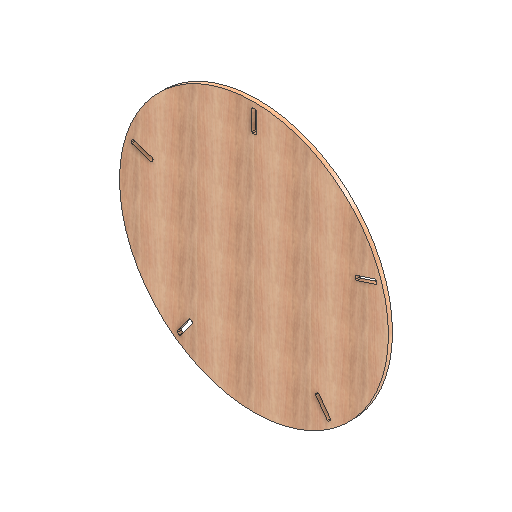
# Autodesk Inventor part: Disk G
Saved by Autodesk Inventor 2021 (Build 250183000, 183)
## iProperties
Created: 2020-05-09
Part Number: Disk G
Material: Wood (Birch)
Document SubType Name: Modeling
Designer: Dan Wikman
Density: 0.55 g/cm^3
Appearance: Birch - Natural Polished
Mass: 11105 g
Surface Area: 23317.4 cm^2
Volume: 20191 cm^3
Autodesk Inventor part; units mm, degrees
ref_plane "YZ Plane" through (0, 0, 0) normal (1, 0, 0) x (0, 1, 0)
ref_plane "XZ Plane" through (0, 0, 0) normal (0, 1, 0) x (-1, 0, 0)
ref_plane "XY Plane" through (0, 0, 0) normal (0, 0, 1) x (1, 0, 0)
sketch "CONTOURS" plane through (0, 0, 0) normal (0, 0, 1) x (1, 0, 0)
  circle A0 centre (614.9903, 609.9576) radius 599.9973
  dimension "d3" = 1199.9946
  constraints: 1 centre point
  measures "d3" diameter of A0
sketch "HOLES" plane through (0, 0, 0) normal (0, 0, 1) x (1, 0, 0)
  line L0 (1162.6152, 782.0631) -> (1159.216, 792.5247)
  arc A0 (1159.216, 792.5247) -> (1154.1757, 795.0928) centre (1155.4118, 791.2886) ccw
  line L1 (1154.1757, 795.0928) -> (1068.5806, 767.2813)
  arc A1 (1068.5806, 767.2813) -> (1066.0124, 762.241) centre (1069.8167, 763.4771) ccw
  line L2 (1066.0124, 762.241) -> (1069.4116, 751.7794)
  arc A2 (1069.4116, 751.7794) -> (1074.4519, 749.2112) centre (1073.2159, 753.0155) ccw
  line L3 (1074.4519, 749.2112) -> (1160.047, 777.0228)
  arc A3 (1160.047, 777.0228) -> (1162.6152, 782.0631) centre (1158.8109, 780.827) ccw
  line L4 (947.8978, 142.3189) -> (956.7969, 148.7846)
  arc A4 (956.7969, 148.7846) -> (957.6819, 154.3718) centre (954.4458, 152.0206) ccw
  line L5 (957.6819, 154.3718) -> (904.7812, 227.1833)
  arc A5 (904.7812, 227.1833) -> (899.194, 228.0682) centre (901.5451, 224.8322) ccw
  line L6 (899.194, 228.0682) -> (890.2948, 221.6026)
  arc A6 (890.2948, 221.6026) -> (889.4099, 216.0154) centre (892.6459, 218.3665) ccw
  line L7 (889.4099, 216.0154) -> (942.3106, 143.2039)
  arc A7 (942.3106, 143.2039) -> (947.8978, 142.3189) centre (945.5466, 145.555) ccw
  line L8 (620.5337, 1183.9633) -> (609.5337, 1183.9633)
  arc A8 (609.5337, 1183.9633) -> (605.5337, 1179.9633) centre (609.5337, 1179.9633) ccw
  line L9 (605.5337, 1179.9633) -> (605.5337, 1089.9633)
  arc A9 (605.5337, 1089.9633) -> (609.5337, 1085.9633) centre (609.5337, 1089.9633) ccw
  line L10 (609.5337, 1085.9633) -> (620.5337, 1085.9633)
  arc A10 (620.5337, 1085.9633) -> (624.5337, 1089.9633) centre (620.5337, 1089.9633) ccw
  line L11 (624.5337, 1089.9633) -> (624.5337, 1179.9633)
  arc A11 (624.5337, 1179.9633) -> (620.5337, 1183.9633) centre (620.5337, 1179.9633) ccw
  line L12 (273.1136, 148.8355) -> (282.0128, 142.3699)
  arc A12 (282.0128, 142.3699) -> (287.6, 143.2548) centre (284.3639, 145.6059) ccw
  line L13 (287.6, 143.2548) -> (340.5007, 216.0663)
  arc A13 (340.5007, 216.0663) -> (339.6157, 221.6535) centre (337.2646, 218.4175) ccw
  line L14 (339.6157, 221.6535) -> (330.7166, 228.1192)
  arc A14 (330.7166, 228.1192) -> (325.1293, 227.2342) centre (328.3654, 224.8831) ccw
  line L15 (325.1293, 227.2342) -> (272.2287, 154.4227)
  arc A15 (272.2287, 154.4227) -> (273.1136, 148.8355) centre (275.4647, 152.0716) ccw
  line L16 (70.7915, 792.6071) -> (67.3923, 782.1455)
  arc A16 (67.3923, 782.1455) -> (69.9604, 777.1052) centre (71.1965, 780.9094) ccw
  line L17 (69.9604, 777.1052) -> (155.5555, 749.2937)
  arc A17 (155.5555, 749.2937) -> (160.5958, 751.8618) centre (156.7916, 753.0979) ccw
  line L18 (160.5958, 751.8618) -> (163.995, 762.3235)
  arc A18 (163.995, 762.3235) -> (161.4268, 767.3637) centre (160.1908, 763.5595) ccw
  line L19 (161.4268, 767.3637) -> (75.8318, 795.1753)
  arc A19 (75.8318, 795.1753) -> (70.7915, 792.6071) centre (74.5957, 791.371) ccw
  dimension "d1" = 19
  dimension "d19" = 90
  constraints: 40 end point, 40 point on circle, 20 centre point
  measures "d1" distance of L9.start L11.end
  measures "d19" distance of L11.start L11.end
sketch "LETTERS" plane through (0, 0, 0) normal (0, 0, 1) x (1, 0, 0)
  line L0 (622.9768, 614.1235) -> (622.8555, 614.5546)
  line L1 (622.8555, 614.5546) -> (622.7333, 614.956)
  line L2 (622.7333, 614.956) -> (622.6101, 615.3276)
  line L3 (622.6101, 615.3276) -> (622.4861, 615.6694)
  line L4 (622.4861, 615.6694) -> (622.4237, 615.8291)
  line L5 (622.4237, 615.8291) -> (622.3611, 615.9814)
  line L6 (622.3611, 615.9814) -> (622.2982, 616.1262)
  line L7 (622.2982, 616.1262) -> (622.2351, 616.2636)
  line L8 (622.2351, 616.2636) -> (622.1718, 616.3935)
  line L9 (622.1718, 616.3935) -> (622.1083, 616.516)
  line L10 (622.1083, 616.516) -> (622.0445, 616.631)
  line L11 (622.0445, 616.631) -> (621.9805, 616.7386)
  line L12 (621.9805, 616.7386) -> (621.9154, 616.8417)
  line L13 (621.9154, 616.8417) -> (621.8484, 616.943)
  line L14 (621.8484, 616.943) -> (621.7795, 617.0428)
  line L15 (621.7795, 617.0428) -> (621.7087, 617.1408)
  line L16 (621.7087, 617.1408) -> (621.6361, 617.2373)
  line L17 (621.6361, 617.2373) -> (621.5615, 617.3321)
  line L18 (621.5615, 617.3321) -> (621.485, 617.4252)
  line L19 (621.485, 617.4252) -> (621.4066, 617.5167)
  line L20 (621.4066, 617.5167) -> (621.3264, 617.6065)
  line L21 (621.3264, 617.6065) -> (621.2442, 617.6947)
  line L22 (621.2442, 617.6947) -> (621.1602, 617.7812)
  line L23 (621.1602, 617.7812) -> (621.0742, 617.8661)
  line L24 (621.0742, 617.8661) -> (620.9864, 617.9494)
  line L25 (620.9864, 617.9494) -> (620.8966, 618.031)
  line L26 (620.8966, 618.031) -> (620.805, 618.1109)
  line L27 (620.805, 618.1109) -> (620.7115, 618.1892)
  line L28 (620.7115, 618.1892) -> (620.5209, 618.3409)
  line L29 (620.5209, 618.3409) -> (620.3269, 618.4859)
  line L30 (620.3269, 618.4859) -> (620.1297, 618.6242)
  line L31 (620.1297, 618.6242) -> (619.9292, 618.756)
  line L32 (619.9292, 618.756) -> (619.7254, 618.8811)
  line L33 (619.7254, 618.8811) -> (619.5183, 618.9995)
  line L34 (619.5183, 618.9995) -> (619.3079, 619.1114)
  line L35 (619.3079, 619.1114) -> (619.0942, 619.2166)
  line L36 (619.0942, 619.2166) -> (618.9858, 619.2666)
  line L37 (618.9858, 619.2666) -> (618.8761, 619.3148)
  line L38 (618.8761, 619.3148) -> (618.765, 619.3612)
  line L39 (618.765, 619.3612) -> (618.6526, 619.4058)
  line L40 (618.6526, 619.4058) -> (618.5388, 619.4485)
  line L41 (618.5388, 619.4485) -> (618.4237, 619.4895)
  line L42 (618.4237, 619.4895) -> (618.3072, 619.5286)
  line L43 (618.3072, 619.5286) -> (618.1894, 619.5658)
  line L44 (618.1894, 619.5658) -> (617.9497, 619.6349)
  line L45 (617.9497, 619.6349) -> (617.7046, 619.6967)
  line L46 (617.7046, 619.6967) -> (617.454, 619.7512)
  line L47 (617.454, 619.7512) -> (617.1981, 619.7984)
  line L48 (617.1981, 619.7984) -> (616.9346, 619.8392)
  line L49 (616.9346, 619.8392) -> (616.6613, 619.8746)
  line L50 (616.6613, 619.8746) -> (616.3784, 619.9045)
  line L51 (616.3784, 619.9045) -> (616.0858, 619.929)
  line L52 (616.0858, 619.929) -> (615.7835, 619.9481)
  line L53 (615.7835, 619.9481) -> (615.4715, 619.9617)
  line L54 (615.4715, 619.9617) -> (614.8184, 619.9726)
  line L55 (614.8184, 619.9726) -> (614.1719, 619.964)
  line L56 (614.1719, 619.964) -> (613.5774, 619.9385)
  line L57 (613.5774, 619.9385) -> (613.2996, 619.9194)
  line L58 (613.2996, 619.9194) -> (613.0349, 619.8959)
  line L59 (613.0349, 619.8959) -> (612.7831, 619.8683)
  line L60 (612.7831, 619.8683) -> (612.5443, 619.8364)
  line L61 (612.5443, 619.8364) -> (612.3121, 619.7985)
  line L62 (612.3121, 619.7985) -> (612.0798, 619.7532)
  line L63 (612.0798, 619.7532) -> (611.8476, 619.7002)
  line L64 (611.8476, 619.7002) -> (611.6153, 619.6397)
  line L65 (611.6153, 619.6397) -> (611.383, 619.5717)
  line L66 (611.383, 619.5717) -> (611.1508, 619.4961)
  line L67 (611.1508, 619.4961) -> (610.9185, 619.4129)
  line L68 (610.9185, 619.4129) -> (610.6862, 619.3222)
  line L69 (610.6862, 619.3222) -> (610.4529, 619.2229)
  line L70 (610.4529, 619.2229) -> (610.2174, 619.1139)
  line L71 (610.2174, 619.1139) -> (609.9798, 618.9952)
  line L72 (609.9798, 618.9952) -> (609.74, 618.8669)
  line L73 (609.74, 618.8669) -> (609.4981, 618.7289)
  line L74 (609.4981, 618.7289) -> (609.2541, 618.5813)
  line L75 (609.2541, 618.5813) -> (609.0078, 618.424)
  line L76 (609.0078, 618.424) -> (608.7595, 618.257)
  line L77 (608.7595, 618.257) -> (608.6356, 618.1697)
  line L78 (608.6356, 618.1697) -> (608.5134, 618.0797)
  line L79 (608.5134, 618.0797) -> (608.3928, 617.987)
  line L80 (608.3928, 617.987) -> (608.2739, 617.8916)
  line L81 (608.2739, 617.8916) -> (608.1567, 617.7935)
  line L82 (608.1567, 617.7935) -> (608.0411, 617.6927)
  line L83 (608.0411, 617.6927) -> (607.9272, 617.5891)
  line L84 (607.9272, 617.5891) -> (607.8149, 617.4828)
  line L85 (607.8149, 617.4828) -> (607.7043, 617.3739)
  line L86 (607.7043, 617.3739) -> (607.5953, 617.2622)
  line L87 (607.5953, 617.2622) -> (607.488, 617.1478)
  line L88 (607.488, 617.1478) -> (607.3824, 617.0307)
  line L89 (607.3824, 617.0307) -> (607.2784, 616.9108)
  line L90 (607.2784, 616.9108) -> (607.176, 616.7883)
  line L91 (607.176, 616.7883) -> (607.0754, 616.663)
  line L92 (607.0754, 616.663) -> (606.9764, 616.5351)
  line L93 (606.9764, 616.5351) -> (606.8795, 616.4051)
  line L94 (606.8795, 616.4051) -> (606.7852, 616.2738)
  line L95 (618.3393, 599.944) -> (618.5538, 599.9977)
  line L96 (618.5538, 599.9977) -> (618.7672, 600.0568)
  line L97 (618.7672, 600.0568) -> (618.9794, 600.1214)
  line L98 (618.9794, 600.1214) -> (619.1905, 600.1913)
  line L99 (619.1905, 600.1913) -> (619.4004, 600.2667)
  line L100 (619.4004, 600.2667) -> (619.6092, 600.3476)
  line L101 (619.6092, 600.3476) -> (619.8168, 600.4339)
  line L102 (619.8168, 600.4339) -> (620.0233, 600.5256)
  line L103 (620.0233, 600.5256) -> (620.2287, 600.6223)
  line L104 (620.2287, 600.6223) -> (620.4332, 600.7235)
  line L105 (620.4332, 600.7235) -> (620.6368, 600.8291)
  line L106 (620.6368, 600.8291) -> (620.8394, 600.9391)
  line L107 (620.8394, 600.9391) -> (621.0411, 601.0536)
  line L108 (621.0411, 601.0536) -> (621.2419, 601.1726)
  line L109 (621.2419, 601.1726) -> (621.4418, 601.296)
  line L110 (621.4418, 601.296) -> (621.6408, 601.4239)
  line L111 (621.6408, 601.4239) -> (622.3722, 601.9163)
  line L112 (622.3722, 601.9163) -> (622.691, 602.1415)
  line L113 (622.691, 602.1415) -> (622.9785, 602.3528)
  line L114 (622.9785, 602.3528) -> (623.4053, 602.6781)
  line L115 (623.4053, 602.6781) -> (623.5311, 602.7785)
  line L116 (623.5311, 602.7785) -> (623.572, 602.8131)
  line L117 (605.8556, 614.5967) -> (605.795, 614.4485)
  line L118 (623.587, 602.8265) -> (623.5931, 602.8322)
  line L119 (623.5931, 602.8322) -> (623.5983, 602.8373)
  line L120 (623.5983, 602.8373) -> (623.5992, 609.9994)
  line L121 (623.5992, 609.9994) -> (615.0012, 610.0005)
  line L122 (605.7369, 614.299) -> (605.5299, 613.7237)
  line L123 (605.5299, 613.7237) -> (605.4413, 613.4552)
  line L124 (605.4413, 613.4552) -> (605.3626, 613.1994)
  line L125 (605.3626, 613.1994) -> (605.294, 612.9564)
  line L126 (605.294, 612.9564) -> (605.2353, 612.7261)
  line L127 (605.2353, 612.7261) -> (605.1866, 612.5085)
  line L128 (605.1866, 612.5085) -> (605.1659, 612.4045)
  line L129 (605.1659, 612.4045) -> (605.1478, 612.3036)
  line L130 (605.1478, 612.3036) -> (605.0844, 611.8916)
  line L131 (605.0844, 611.8916) -> (605.0293, 611.4495)
  line L132 (605.0293, 611.4495) -> (604.9825, 610.9774)
  line L133 (604.9825, 610.9774) -> (604.944, 610.4751)
  line L134 (604.944, 610.4751) -> (604.9301, 610.2143)
  line L135 (604.9301, 610.2143) -> (604.9225, 609.9493)
  line L136 (604.9225, 609.9493) -> (604.9214, 609.68)
  line L137 (604.9214, 609.68) -> (604.9266, 609.4064)
  line L138 (604.9266, 609.4064) -> (604.9383, 609.1286)
  line L139 (604.9383, 609.1286) -> (604.9563, 608.8465)
  line L140 (604.9563, 608.8465) -> (604.9808, 608.5602)
  line L141 (604.9808, 608.5602) -> (605.0116, 608.2696)
  line L142 (605.0116, 608.2696) -> (605.049, 607.9781)
  line L143 (605.049, 607.9781) -> (605.0929, 607.6889)
  line L144 (605.0929, 607.6889) -> (605.1434, 607.4021)
  line L145 (605.1434, 607.4021) -> (605.2006, 607.1176)
  line L146 (605.2006, 607.1176) -> (605.2643, 606.8354)
  line L147 (605.2643, 606.8354) -> (605.3347, 606.5556)
  line L148 (605.3347, 606.5556) -> (605.4116, 606.2781)
  line L149 (605.4116, 606.2781) -> (605.4951, 606.003)
  line L150 (605.4951, 606.003) -> (605.5846, 605.7331)
  line L151 (605.5846, 605.7331) -> (605.6792, 605.4716)
  line L152 (605.6792, 605.4716) -> (605.7791, 605.2183)
  line L153 (605.7791, 605.2183) -> (605.8842, 604.9733)
  line L154 (605.8842, 604.9733) -> (605.9945, 604.7366)
  line L155 (605.9945, 604.7366) -> (606.11, 604.5082)
  line L156 (606.11, 604.5082) -> (606.2307, 604.2881)
  line L157 (606.2307, 604.2881) -> (606.293, 604.1811)
  line L158 (606.293, 604.1811) -> (606.3566, 604.0762)
  line L159 (606.3566, 604.0762) -> (606.4874, 603.8703)
  line L160 (606.4874, 603.8703) -> (606.6226, 603.6678)
  line L161 (606.6226, 603.6678) -> (606.7623, 603.469)
  line L162 (606.7623, 603.469) -> (606.9064, 603.2736)
  line L163 (606.9064, 603.2736) -> (607.055, 603.0818)
  line L164 (607.055, 603.0818) -> (607.208, 602.8935)
  line L165 (607.208, 602.8935) -> (607.3655, 602.7087)
  line L166 (607.3655, 602.7087) -> (607.5275, 602.5274)
  line L167 (607.5275, 602.5274) -> (607.6932, 602.351)
  line L168 (605.795, 614.4485) -> (605.7369, 614.299)
  line L169 (607.6932, 602.351) -> (607.862, 602.1808)
  line L170 (607.862, 602.1808) -> (608.0339, 602.0166)
  line L171 (608.0339, 602.0166) -> (608.2089, 601.8586)
  line L172 (608.2089, 601.8586) -> (608.3871, 601.7068)
  line L173 (608.3871, 601.7068) -> (608.5683, 601.561)
  line L174 (608.5683, 601.561) -> (608.7526, 601.4215)
  line L175 (608.7526, 601.4215) -> (608.94, 601.288)
  line L176 (608.94, 601.288) -> (609.1322, 601.1594)
  line L177 (609.1322, 601.1594) -> (609.3307, 601.0344)
  line L178 (609.3307, 601.0344) -> (609.5356, 600.9129)
  line L179 (609.5356, 600.9129) -> (609.7469, 600.795)
  line L180 (609.7469, 600.795) -> (609.9645, 600.6806)
  line L181 (609.9645, 600.6806) -> (610.1885, 600.5698)
  line L182 (610.1885, 600.5698) -> (610.4189, 600.4626)
  line L183 (610.4189, 600.4626) -> (610.6556, 600.359)
  line L184 (610.6556, 600.359) -> (610.8962, 600.2607)
  line L185 (610.8962, 600.2607) -> (611.1383, 600.1698)
  line L186 (611.1383, 600.1698) -> (611.3818, 600.0861)
  line L187 (611.3818, 600.0861) -> (611.6266, 600.0098)
  line L188 (611.6266, 600.0098) -> (611.8729, 599.9407)
  line L189 (611.8729, 599.9407) -> (612.1207, 599.8789)
  line L190 (612.1207, 599.8789) -> (612.3698, 599.8244)
  line L191 (612.3698, 599.8244) -> (612.6204, 599.7772)
  line L192 (612.6204, 599.7772) -> (613.1224, 599.6968)
  line L193 (613.1224, 599.6968) -> (613.6233, 599.6297)
  line L194 (613.6233, 599.6297) -> (614.1232, 599.5759)
  line L195 (614.1232, 599.5759) -> (614.622, 599.5355)
  line L196 (614.622, 599.5355) -> (614.8702, 599.5218)
  line L197 (614.8702, 599.5218) -> (615.1162, 599.5144)
  line L198 (615.1162, 599.5144) -> (615.3602, 599.5135)
  line L199 (615.3602, 599.5135) -> (615.602, 599.5188)
  line L200 (615.602, 599.5188) -> (615.8418, 599.5306)
  line L201 (615.8418, 599.5306) -> (616.0796, 599.5487)
  line L202 (616.0796, 599.5487) -> (616.3152, 599.5732)
  line L203 (616.3152, 599.5732) -> (616.5488, 599.6041)
  line L204 (616.5488, 599.6041) -> (617.0095, 599.6764)
  line L205 (617.0095, 599.6764) -> (617.4615, 599.7572)
  line L206 (617.4615, 599.7572) -> (617.9047, 599.8464)
  line L207 (617.9047, 599.8464) -> (618.3393, 599.944)
  line L208 (605.9188, 614.7437) -> (605.8556, 614.5967)
  line L209 (605.9846, 614.8893) -> (605.9188, 614.7437)
  line L210 (606.053, 615.0336) -> (605.9846, 614.8893)
  line L211 (606.124, 615.1766) -> (606.053, 615.0336)
  line L212 (606.1976, 615.3183) -> (606.124, 615.1766)
  line L213 (606.2738, 615.4587) -> (606.1976, 615.3183)
  line L214 (606.3525, 615.5978) -> (606.2738, 615.4587)
  line L215 (606.4339, 615.7356) -> (606.3525, 615.5978)
  line L216 (606.5178, 615.8721) -> (606.4339, 615.7356)
  line L217 (606.6043, 616.0073) -> (606.5178, 615.8721)
  line L218 (606.6935, 616.1412) -> (606.6043, 616.0073)
  line L219 (606.7852, 616.2738) -> (606.6935, 616.1412)
  line L220 (623.572, 602.8131) -> (623.587, 602.8265)
  constraints: 442 end point, 3 parallel, 2 perpendicular
extrude "Extrusion4" add sketch "CONTOURS" along normal blind 18
extrude "Extrusion5" cut sketch "HOLES" along normal blind 18
body "Solid2"
